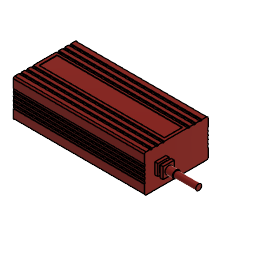
SSRHeatsink (Autodesk Fusion 360 archive; units mm, degrees)
design "BatteryCharger"
part number: 2026-09-24-16-56-48-668
Autodesk Fusion 360 part; units mm, degrees
note: some values were not read from the file. Set by a fixed rule: which face or edge a step refers to.
(part 1 of 3)
sketch "Sketch1" plane through (0, 0, 0) normal (0, 0, 1) x (1, 0, 0)
  line L0 (-87.5, 42.5) -> (87.5, 42.5)
  line L1 (87.5, 42.5) -> (87.5, -42.5)
  line L2 (87.5, -42.5) -> (-87.5, -42.5)
  line L3 (-87.5, -42.5) -> (-87.5, 42.5)
  line L4 (-87.5, 42.5) -> (87.5, -42.5) construction
  line L5 (87.5, 42.5) -> (-87.5, -42.5) construction
  dimension "d1" = 175
  dimension "d2" = 85
  constraint horizontal L0
  constraint perpendicular L0 L1
  constraint parallel L0 L2
  constraint parallel L1 L3
  constraint coincident L4 origin
  constraint coincident L5 origin
  measures "d1" distance of L1.end L2.end
  measures "d2" distance of L0.end L1.end
extrude "Extrude1" add sketch "Sketch1" along normal blind 50
sketch "Sketch2" plane through (0, 0, 50) normal (0, 0, 1) x (-1, 0, 0)
  line L0 (87.5, 42.5) -> (-87.5, 42.5)
  line L1 (-87.5, 42.5) -> (-87.5, -42.5)
  line L2 (-87.5, -42.5) -> (87.5, -42.5)
  line L3 (87.5, -42.5) -> (87.5, 42.5)
  line L4 (87.5, -15) -> (-87.5, -15)
  line L5 (-87.5, -15) -> (-87.5, 15)
  line L6 (-87.5, 15) -> (87.5, 15)
  line L7 (87.5, 15) -> (87.5, -15)
  line L8 (87.5, -15) -> (-87.5, 15) construction
  line L9 (-87.5, -15) -> (87.5, 15) construction
  line L10 (87.5, -15) -> (-87.5, -15)
  line L11 (-87.5, -15) -> (-87.5, -18)
  line L12 (-87.5, -18) -> (87.5, -18)
  line L13 (87.5, -18) -> (87.5, -15)
  line L14 (87.5, -18) -> (-87.5, -18)
  line L15 (-87.5, -18) -> (-87.5, -23)
  line L16 (-87.5, -23) -> (87.5, -23)
  line L17 (87.5, -23) -> (87.5, -18)
  line L18 (87.5, -23) -> (-87.5, -23)
  line L19 (-87.5, -23) -> (-87.5, -26)
  line L20 (-87.5, -26) -> (87.5, -26)
  line L21 (87.5, -26) -> (87.5, -23)
  line L22 (87.5, -26) -> (-87.5, -26)
  line L23 (-87.5, -26) -> (-87.5, -31)
  line L24 (-87.5, -31) -> (87.5, -31)
  line L25 (87.5, -31) -> (87.5, -26)
  line L26 (87.5, -31) -> (-87.5, -31)
  line L27 (-87.5, -31) -> (-87.5, -34)
  line L28 (-87.5, -34) -> (87.5, -34)
  line L29 (87.5, -34) -> (87.5, -31)
  dimension "d5" = 30
  dimension "d6" = 3
  dimension "d7" = 5
  dimension "d8" = 3
  dimension "d9" = 5
  dimension "d10" = 3
  constraint horizontal L4
  constraint perpendicular L4 L5
  constraint parallel L4 L6
  constraint parallel L5 L7
  constraint coincident L8 origin
  constraint coincident L9 origin
  constraint horizontal L10
  constraint vertical L11
  constraint horizontal L12
  constraint vertical L13
  constraint horizontal L14
  constraint vertical L15
  constraint horizontal L16
  constraint vertical L17
  constraint horizontal L18
  constraint vertical L19
  constraint horizontal L20
  constraint vertical L21
  constraint horizontal L22
  constraint vertical L23
  constraint horizontal L24
  constraint vertical L25
  constraint horizontal L26
  constraint vertical L27
  constraint horizontal L28
  constraint vertical L29
  measures "d5" distance of L4.end L5.end
  measures "d6" distance of L4.start L12.end
  measures "d7" distance of L12.end L16.end
  measures "d8" distance of L16.end L20.end
  measures "d9" distance of L20.end L24.end
  measures "d10" distance of L24.end L28.end
extrude "Extrude2" cut sketch "Sketch2" against normal blind 0.5 contours L1 L3 L4 L10 L11 L12 L13 L14 | L1 L3 L16 L18 L19 L20 L21 L22 | L1 L3 L24 L26 L27 L28 L29
fillet "Fillet1" radius 0.5 3 faces at (29.1667, 32, 49.5) (29.1667, 25, 49.5) (-29.1667, 16, 49.5)
pattern_linear "R-Pattern1" count 1 spacing 0 along (1, 0, 0) count 2 spacing 50 along (0, -1, 0) of "Extrude2", "Fillet1"
sketch "Sketch3" plane through (0, 0, 50) normal (0, 0, 1) x (-1, 0, 0)
  line L0 (87.5, 16) -> (87, 16)
  line L1 (87, 16) -> (-87, 16)
  line L2 (-87, 16) -> (-87.5, 16)
  line L3 (-87.5, 16) -> (-87.5, -15)
  line L4 (-87.5, -15) -> (-87, -15)
  line L5 (-87, -15) -> (87, -15)
  line L6 (87, -15) -> (87.5, -15)
  line L7 (87.5, -15) -> (87.5, 16)
  line L8 (83.4341, -11.9471) -> (-83.4341, -11.9471)
  line L9 (-83.4341, -11.9471) -> (-83.4341, 11.9471)
  line L10 (-83.4341, 11.9471) -> (83.4341, 11.9471)
  line L11 (83.4341, 11.9471) -> (83.4341, -11.9471)
  line L12 (83.4341, -11.9471) -> (-83.4341, 11.9471) construction
  line L13 (-83.4341, -11.9471) -> (83.4341, 11.9471) construction
  constraint horizontal L8
  constraint perpendicular L8 L9
  constraint parallel L8 L10
  constraint parallel L9 L11
  constraint coincident L12 origin
  constraint coincident L13 origin
extrude "Extrude3" cut sketch "Sketch3" against normal blind 0.5 contours L8 L9 L10 L11
sketch "Sketch4" plane through (0, -42.5, 0) normal (0, -1, 0) x (1, 0, 0)
  line L0 (-87.5, 0) -> (87.5, 0)
  line L1 (87.5, 0) -> (87.5, 50)
  line L2 (87.5, 50) -> (-87.5, 50)
  line L3 (-87.5, 50) -> (-87.5, 0)
  line L4 (0, 50) -> (0, 0) construction
  line L5 (-87.5, 26.5) -> (87.5, 26.5)
  line L6 (87.5, 26.5) -> (87.5, 23.5)
  line L7 (87.5, 23.5) -> (-87.5, 23.5)
  line L8 (-87.5, 23.5) -> (-87.5, 26.5)
  line L9 (-87.5, 26.5) -> (87.5, 23.5) construction
  line L10 (87.5, 26.5) -> (-87.5, 23.5) construction
  point P0 (0, 25)
  dimension "d21" = 3
  constraint midpoint L2 L4.start
  constraint coincident L4.end origin
  constraint horizontal L5
  constraint perpendicular L5 L6
  constraint parallel L5 L7
  constraint parallel L6 L8
  constraint coincident L9 P0
  constraint coincident L10 P0
  constraint midpoint L4 P0
  measures "d21" distance of L5.end L6.end
extrude "Extrude4" cut sketch "Sketch4" against normal blind 0.5 contours L1 L3 L5 L6 L7 L8
pattern_linear "R-Pattern2" count 1 spacing 0 along (-1, 0, 0) count 5 spacing 5 along (0, 0, 1) both ways of "Extrude4"
pattern_linear "R-Pattern3" count 1 spacing 0 along (0, 0, -1) count 2 spacing 84.5 along (0, 1, 0) of "Extrude4", "R-Pattern2"
fillet "Fillet2" radius 2 4 edges at (0, 42.5, 50) (0, 42.5, 0) (0, -42.5, 0) (0, -42.5, 50)
sketch "Sketch5" plane through (-87.5, 0, 0) normal (-1, 0, 0) x (0, -1, 0)
  arc A0 (42.5, 48) -> (40.5, 50) centre (40.5, 48) ccw
  line L0 (40.5, 50) -> (35, 50)
  line L1 (35, 50) -> (35, 49.866)
  spline S0 degree 3 poles (34.5, 49) (34.6385, 49.1385) (34.802, 49.3076) (34.9552, 49.5924) (35, 49.7386) (35, 49.866) knots 0 0 0 0 0.058781 0.058781 0.097013 0.097013 0.097013 0.097013
  line L2 (34.5, 49) -> (32.5, 49)
  spline S1 degree 3 poles (32, 49.866) (32, 49.7386) (32.0448, 49.5924) (32.198, 49.3076) (32.3615, 49.1385) (32.5, 49) knots 0.252766 0.252766 0.252766 0.252766 0.290998 0.290998 0.349779 0.349779 0.349779 0.349779
  line L3 (32, 49.866) -> (32, 50)
  line L4 (32, 50) -> (27, 50)
  line L5 (27, 50) -> (27, 49.866)
  spline S2 degree 3 poles (26.5, 49) (26.6385, 49.1385) (26.802, 49.3076) (26.9552, 49.5924) (27, 49.7386) (27, 49.866) knots 0 0 0 0 0.058781 0.058781 0.097013 0.097013 0.097013 0.097013
  line L6 (26.5, 49) -> (24.5, 49)
  spline S3 degree 3 poles (24, 49.866) (24, 49.7386) (24.0448, 49.5924) (24.198, 49.3076) (24.3615, 49.1385) (24.5, 49) knots 0.252766 0.252766 0.252766 0.252766 0.290998 0.290998 0.349779 0.349779 0.349779 0.349779
  line L7 (24, 49.866) -> (24, 50)
  line L8 (24, 50) -> (19, 50)
  line L9 (19, 50) -> (19, 49.866)
  spline S4 degree 3 poles (18.5, 49) (18.6385, 49.1385) (18.802, 49.3076) (18.9552, 49.5924) (19, 49.7386) (19, 49.866) knots 0 0 0 0 0.058781 0.058781 0.097013 0.097013 0.097013 0.097013
  line L10 (18.5, 49) -> (16.5, 49)
  spline S5 degree 3 poles (16, 49.866) (16, 49.7386) (16.0448, 49.5924) (16.198, 49.3076) (16.3615, 49.1385) (16.5, 49) knots 0.252766 0.252766 0.252766 0.252766 0.290998 0.290998 0.349779 0.349779 0.349779 0.349779
  line L11 (16, 49.866) -> (16, 50)
  line L12 (16, 50) -> (-15, 50)
  line L13 (-15, 50) -> (-15, 49.866)
  spline S6 degree 3 poles (-15.5, 49) (-15.3615, 49.1385) (-15.198, 49.3076) (-15.0448, 49.5924) (-15, 49.7386) (-15, 49.866) knots 0 0 0 0 0.058781 0.058781 0.097013 0.097013 0.097013 0.097013
  line L14 (-15.5, 49) -> (-17.5, 49)
  spline S7 degree 3 poles (-18, 49.866) (-18, 49.7386) (-17.9552, 49.5924) (-17.802, 49.3076) (-17.6385, 49.1385) (-17.5, 49) knots 0.252766 0.252766 0.252766 0.252766 0.290998 0.290998 0.349779 0.349779 0.349779 0.349779
  line L15 (-18, 49.866) -> (-18, 50)
  line L16 (-18, 50) -> (-23, 50)
  line L17 (-23, 50) -> (-23, 49.866)
  spline S8 degree 3 poles (-23.5, 49) (-23.3615, 49.1385) (-23.198, 49.3076) (-23.0448, 49.5924) (-23, 49.7386) (-23, 49.866) knots 0 0 0 0 0.058781 0.058781 0.097013 0.097013 0.097013 0.097013
  line L18 (-23.5, 49) -> (-25.5, 49)
  spline S9 degree 3 poles (-26, 49.866) (-26, 49.7386) (-25.9552, 49.5924) (-25.802, 49.3076) (-25.6385, 49.1385) (-25.5, 49) knots 0.252766 0.252766 0.252766 0.252766 0.290998 0.290998 0.349779 0.349779 0.349779 0.349779
  line L19 (-26, 49.866) -> (-26, 50)
  line L20 (-26, 50) -> (-31, 50)
  line L21 (-31, 50) -> (-31, 49.866)
  spline S10 degree 3 poles (-31.5, 49) (-31.3615, 49.1385) (-31.198, 49.3076) (-31.0448, 49.5924) (-31, 49.7386) (-31, 49.866) knots 0 0 0 0 0.058781 0.058781 0.097013 0.097013 0.097013 0.097013
  line L22 (-31.5, 49) -> (-33.5, 49)
  spline S11 degree 3 poles (-34, 49.866) (-34, 49.7386) (-33.9552, 49.5924) (-33.802, 49.3076) (-33.6385, 49.1385) (-33.5, 49) knots 0.252766 0.252766 0.252766 0.252766 0.290998 0.290998 0.349779 0.349779 0.349779 0.349779
  line L23 (-34, 49.866) -> (-34, 50)
  line L24 (-34, 50) -> (-40.5, 50)
  arc A1 (-40.5, 50) -> (-42.5, 48) centre (-40.5, 48) ccw
  line L25 (-42.5, 48) -> (-42.5, 36.5)
  line L26 (-42.5, 36.5) -> (-42, 36.5)
  line L27 (-42, 36.5) -> (-42, 33.5)
  line L28 (-42, 33.5) -> (-42.5, 33.5)
  line L29 (-42.5, 33.5) -> (-42.5, 31.5)
  line L30 (-42.5, 31.5) -> (-42, 31.5)
  line L31 (-42, 31.5) -> (-42, 28.5)
  line L32 (-42, 28.5) -> (-42.5, 28.5)
  line L33 (-42.5, 28.5) -> (-42.5, 26.5)
  line L34 (-42.5, 26.5) -> (-42, 26.5)
  line L35 (-42, 26.5) -> (-42, 23.5)
  line L36 (-42, 23.5) -> (-42.5, 23.5)
  line L37 (-42.5, 23.5) -> (-42.5, 21.5)
  line L38 (-42.5, 21.5) -> (-42, 21.5)
  line L39 (-42, 21.5) -> (-42, 18.5)
  line L40 (-42, 18.5) -> (-42.5, 18.5)
  line L41 (-42.5, 18.5) -> (-42.5, 16.5)
  line L42 (-42.5, 16.5) -> (-42, 16.5)
  line L43 (-42, 16.5) -> (-42, 13.5)
  line L44 (-42, 13.5) -> (-42.5, 13.5)
  line L45 (-42.5, 13.5) -> (-42.5, 2)
  arc A2 (-42.5, 2) -> (-40.5, 0) centre (-40.5, 2) ccw
  line L46 (-40.5, 0) -> (40.5, 0)
  arc A3 (40.5, 0) -> (42.5, 2) centre (40.5, 2) ccw
  line L47 (42.5, 2) -> (42.5, 13.5)
  line L48 (42.5, 13.5) -> (42, 13.5)
  line L49 (42, 13.5) -> (42, 16.5)
  line L50 (42, 16.5) -> (42.5, 16.5)
  line L51 (42.5, 16.5) -> (42.5, 18.5)
  line L52 (42.5, 18.5) -> (42, 18.5)
  line L53 (42, 18.5) -> (42, 21.5)
  line L54 (42, 21.5) -> (42.5, 21.5)
  line L55 (42.5, 21.5) -> (42.5, 23.5)
  line L56 (42.5, 23.5) -> (42, 23.5)
  line L57 (42, 23.5) -> (42, 26.5)
  line L58 (42, 26.5) -> (42.5, 26.5)
  line L59 (42.5, 26.5) -> (42.5, 28.5)
  line L60 (42.5, 28.5) -> (42, 28.5)
  line L61 (42, 28.5) -> (42, 31.5)
  line L62 (42, 31.5) -> (42.5, 31.5)
  line L63 (42.5, 31.5) -> (42.5, 33.5)
  line L64 (42.5, 33.5) -> (42, 33.5)
  line L65 (42, 33.5) -> (42, 36.5)
  line L66 (42, 36.5) -> (42.5, 36.5)
  line L67 (42.5, 36.5) -> (42.5, 48)
  line L68 (-41.9142, 49.4142) -> (41.9142, 0.5858) construction
  line L69 (-38.5, 45.5) -> (38.5, 45.5) construction
  line L70 (38.5, 45.5) -> (38.5, 4.5) construction
  line L71 (38.5, 4.5) -> (-38.5, 4.5) construction
  line L72 (-38.5, 4.5) -> (-38.5, 45.5) construction
  line L73 (-38.5, 45.5) -> (38.5, 4.5) construction
  line L74 (38.5, 45.5) -> (-38.5, 4.5) construction
  circle A4 centre (-38.5, 45.5) radius 1.5
  circle A5 centre (38.5, 45.5) radius 1.5
  circle A6 centre (-38.5, 4.5) radius 1.5
  circle A7 centre (38.5, 4.5) radius 1.5
  point P0 (0, 25)
  dimension "d34" = 77
  dimension "d35" = 41
  dimension "d36" = 3
  dimension "d37" = 3
  dimension "d38" = 3
  dimension "d39" = 3
  constraint midpoint A1 L68.start
  constraint midpoint A3 L68.end
  constraint horizontal L69
  constraint perpendicular L69 L70
  constraint parallel L69 L71
  constraint parallel L70 L72
  constraint coincident L73 P0
  constraint coincident L74 P0
  constraint midpoint L68 P0
  constraint coincident L69.start L72.end
  constraint coincident L69.end L70.start
  constraint coincident L71.end L72.start
  constraint coincident L70.end L71.start
  measures "d34" distance of L70.end L71.end
  measures "d35" distance of L69.end L70.end
  measures "d36" diameter of A4
  measures "d37" diameter of A5
  measures "d38" diameter of A6
  measures "d39" diameter of A7
extrude "Extrude5" add sketch "Sketch5" along normal blind 2 contours A4 | A5 | A6 | A7
fillet "Fillet3" radius 0.5 4 edges at (-89.5, 39.8985, 44.9576) (-89.5, 39.8985, 3.9576) (-89.5, -37.1015, 44.9576) (-89.5, -37.1015, 3.9576)
sketch "Sketch6" plane through (-87.5, 0, 0) normal (-1, 0, 0) x (0, -1, 0)
  circle A0 centre (38.5, 4.5) radius 1.5
  circle A1 centre (-38.5, 45.5) radius 1.5
  circle A2 centre (38.5, 45.5) radius 1.5
  circle A3 centre (-38.5, 4.5) radius 1.5
  arc A4 (42.5, 48) -> (40.5, 50) centre (40.5, 48) ccw
  line L0 (40.5, 50) -> (35, 50)
  line L1 (35, 50) -> (35, 49.866)
  spline S0 degree 3 poles (34.5, 49) (34.6385, 49.1385) (34.802, 49.3076) (34.9552, 49.5924) (35, 49.7386) (35, 49.866) knots 0 0 0 0 0.058781 0.058781 0.097013 0.097013 0.097013 0.097013
  line L2 (34.5, 49) -> (32.5, 49)
  spline S1 degree 3 poles (32, 49.866) (32, 49.7386) (32.0448, 49.5924) (32.198, 49.3076) (32.3615, 49.1385) (32.5, 49) knots 0.252766 0.252766 0.252766 0.252766 0.290998 0.290998 0.349779 0.349779 0.349779 0.349779
  line L3 (32, 49.866) -> (32, 50)
  line L4 (32, 50) -> (27, 50)
  line L5 (27, 50) -> (27, 49.866)
  spline S2 degree 3 poles (26.5, 49) (26.6385, 49.1385) (26.802, 49.3076) (26.9552, 49.5924) (27, 49.7386) (27, 49.866) knots 0 0 0 0 0.058781 0.058781 0.097013 0.097013 0.097013 0.097013
  line L6 (26.5, 49) -> (24.5, 49)
  spline S3 degree 3 poles (24, 49.866) (24, 49.7386) (24.0448, 49.5924) (24.198, 49.3076) (24.3615, 49.1385) (24.5, 49) knots 0.252766 0.252766 0.252766 0.252766 0.290998 0.290998 0.349779 0.349779 0.349779 0.349779
  line L7 (24, 49.866) -> (24, 50)
  line L8 (24, 50) -> (19, 50)
  line L9 (19, 50) -> (19, 49.866)
  spline S4 degree 3 poles (18.5, 49) (18.6385, 49.1385) (18.802, 49.3076) (18.9552, 49.5924) (19, 49.7386) (19, 49.866) knots 0 0 0 0 0.058781 0.058781 0.097013 0.097013 0.097013 0.097013
  line L10 (18.5, 49) -> (16.5, 49)
  spline S5 degree 3 poles (16, 49.866) (16, 49.7386) (16.0448, 49.5924) (16.198, 49.3076) (16.3615, 49.1385) (16.5, 49) knots 0.252766 0.252766 0.252766 0.252766 0.290998 0.290998 0.349779 0.349779 0.349779 0.349779
  line L11 (16, 49.866) -> (16, 50)
  line L12 (16, 50) -> (-15, 50)
  line L13 (-15, 50) -> (-15, 49.866)
  spline S6 degree 3 poles (-15.5, 49) (-15.3615, 49.1385) (-15.198, 49.3076) (-15.0448, 49.5924) (-15, 49.7386) (-15, 49.866) knots 0 0 0 0 0.058781 0.058781 0.097013 0.097013 0.097013 0.097013
  line L14 (-15.5, 49) -> (-17.5, 49)
  spline S7 degree 3 poles (-18, 49.866) (-18, 49.7386) (-17.9552, 49.5924) (-17.802, 49.3076) (-17.6385, 49.1385) (-17.5, 49) knots 0.252766 0.252766 0.252766 0.252766 0.290998 0.290998 0.349779 0.349779 0.349779 0.349779
  line L15 (-18, 49.866) -> (-18, 50)
  line L16 (-18, 50) -> (-23, 50)
  line L17 (-23, 50) -> (-23, 49.866)
  spline S8 degree 3 poles (-23.5, 49) (-23.3615, 49.1385) (-23.198, 49.3076) (-23.0448, 49.5924) (-23, 49.7386) (-23, 49.866) knots 0 0 0 0 0.058781 0.058781 0.097013 0.097013 0.097013 0.097013
  line L18 (-23.5, 49) -> (-25.5, 49)
  spline S9 degree 3 poles (-26, 49.866) (-26, 49.7386) (-25.9552, 49.5924) (-25.802, 49.3076) (-25.6385, 49.1385) (-25.5, 49) knots 0.252766 0.252766 0.252766 0.252766 0.290998 0.290998 0.349779 0.349779 0.349779 0.349779
  line L19 (-26, 49.866) -> (-26, 50)
  line L20 (-26, 50) -> (-31, 50)
  line L21 (-31, 50) -> (-31, 49.866)
  spline S10 degree 3 poles (-31.5, 49) (-31.3615, 49.1385) (-31.198, 49.3076) (-31.0448, 49.5924) (-31, 49.7386) (-31, 49.866) knots 0 0 0 0 0.058781 0.058781 0.097013 0.097013 0.097013 0.097013
  line L22 (-31.5, 49) -> (-33.5, 49)
  spline S11 degree 3 poles (-34, 49.866) (-34, 49.7386) (-33.9552, 49.5924) (-33.802, 49.3076) (-33.6385, 49.1385) (-33.5, 49) knots 0.252766 0.252766 0.252766 0.252766 0.290998 0.290998 0.349779 0.349779 0.349779 0.349779
  line L23 (-34, 49.866) -> (-34, 50)
  line L24 (-34, 50) -> (-40.5, 50)
  arc A5 (-40.5, 50) -> (-42.5, 48) centre (-40.5, 48) ccw
  line L25 (-42.5, 48) -> (-42.5, 36.5)
  line L26 (-42.5, 36.5) -> (-42, 36.5)
  line L27 (-42, 36.5) -> (-42, 33.5)
  line L28 (-42, 33.5) -> (-42.5, 33.5)
  line L29 (-42.5, 33.5) -> (-42.5, 31.5)
  line L30 (-42.5, 31.5) -> (-42, 31.5)
  line L31 (-42, 31.5) -> (-42, 28.5)
  line L32 (-42, 28.5) -> (-42.5, 28.5)
  line L33 (-42.5, 28.5) -> (-42.5, 26.5)
  line L34 (-42.5, 26.5) -> (-42, 26.5)
  line L35 (-42, 26.5) -> (-42, 23.5)
  line L36 (-42, 23.5) -> (-42.5, 23.5)
  line L37 (-42.5, 23.5) -> (-42.5, 21.5)
  line L38 (-42.5, 21.5) -> (-42, 21.5)
  line L39 (-42, 21.5) -> (-42, 18.5)
  line L40 (-42, 18.5) -> (-42.5, 18.5)
  line L41 (-42.5, 18.5) -> (-42.5, 16.5)
  line L42 (-42.5, 16.5) -> (-42, 16.5)
  line L43 (-42, 16.5) -> (-42, 13.5)
  line L44 (-42, 13.5) -> (-42.5, 13.5)
  line L45 (-42.5, 13.5) -> (-42.5, 2)
  arc A6 (-42.5, 2) -> (-40.5, 0) centre (-40.5, 2) ccw
  line L46 (-40.5, 0) -> (40.5, 0)
  arc A7 (40.5, 0) -> (42.5, 2) centre (40.5, 2) ccw
  line L47 (42.5, 2) -> (42.5, 13.5)
  line L48 (42.5, 13.5) -> (42, 13.5)
  line L49 (42, 13.5) -> (42, 16.5)
  line L50 (42, 16.5) -> (42.5, 16.5)
  line L51 (42.5, 16.5) -> (42.5, 18.5)
  line L52 (42.5, 18.5) -> (42, 18.5)
  line L53 (42, 18.5) -> (42, 21.5)
  line L54 (42, 21.5) -> (42.5, 21.5)
  line L55 (42.5, 21.5) -> (42.5, 23.5)
  line L56 (42.5, 23.5) -> (42, 23.5)
  line L57 (42, 23.5) -> (42, 26.5)
  line L58 (42, 26.5) -> (42.5, 26.5)
  line L59 (42.5, 26.5) -> (42.5, 28.5)
  line L60 (42.5, 28.5) -> (42, 28.5)
  line L61 (42, 28.5) -> (42, 31.5)
  line L62 (42, 31.5) -> (42.5, 31.5)
  line L63 (42.5, 31.5) -> (42.5, 33.5)
  line L64 (42.5, 33.5) -> (42, 33.5)
  line L65 (42, 33.5) -> (42, 36.5)
  line L66 (42, 36.5) -> (42.5, 36.5)
  line L67 (42.5, 36.5) -> (42.5, 48)
  line L68 (42, 25) -> (0, 25) construction
  line L69 (21, 25) -> (-42, 25) construction
  circle A8 centre (-10.5, 25) radius 17.5
  circle A9 centre (-10.5, 25) radius 15
  circle A10 centre (-10.5, 25) radius 12.5
  circle A11 centre (-10.5, 25) radius 10
  circle A12 centre (-10.5, 25) radius 7.5
  line L70 (-9.5, 46.0108) -> (-11.5, 46.0108)
  line L71 (-11.5, 46.0108) -> (-11.5, 3.9892)
  line L72 (-11.5, 3.9892) -> (-9.5, 3.9892)
  line L73 (-9.5, 3.9892) -> (-9.5, 46.0108)
  line L74 (-9.5, 46.0108) -> (-11.5, 3.9892) construction
  line L75 (-11.5, 46.0108) -> (-9.5, 3.9892) construction
  line L76 (15, 26) -> (-36, 26)
  line L77 (-36, 26) -> (-36, 24)
  line L78 (-36, 24) -> (15, 24)
  line L79 (15, 24) -> (15, 26)
  line L80 (15, 26) -> (-36, 24) construction
  line L81 (-36, 26) -> (15, 24) construction
  point P0 (-10.5, 25)
  point P1 (-10.5, 25)
  dimension "d44" = 35
  dimension "d45" = 30
  dimension "d46" = 25
  dimension "d47" = 20
  dimension "d48" = 15
  dimension "d49" = 2
  dimension "d50" = 51
  dimension "d51" = 2
  constraint midpoint L57 L68.start
  constraint perpendicular L57 L68
  constraint midpoint L68 L69.start
  constraint midpoint L35 L69.end
  constraint midpoint L69 P1
  constraint concentric A8 A9
  constraint concentric A8 A10
  constraint concentric A9 A11
  constraint concentric A8 A12
  constraint horizontal L70
  constraint perpendicular L70 L71
  constraint parallel L70 L72
  constraint parallel L71 L73
  constraint coincident L74 P1
  constraint coincident L75 P1
  constraint coincident P1 P0
  constraint horizontal L76
  constraint perpendicular L76 L77
  constraint parallel L76 L78
  constraint parallel L77 L79
  constraint coincident L80 P1
  constraint coincident L81 P1
  measures "d44" diameter of A8
  measures "d45" diameter of A9
  measures "d46" diameter of A10
  measures "d47" diameter of A11
  measures "d48" diameter of A12
  measures "d49" distance of L71.end L72.end
  measures "d50" distance of L77.end L78.end
  measures "d51" distance of L76.end L77.end
extrude "Extrude6" cut sketch "Sketch6" against normal blind 5 contours A8 A9 L73 L76 | A8 A9 L73 L78 | A8 A9 L71 L76 | A10 A11 L73 L76 | A8 A9 L71 L78 | A10 A11 L73 L78 | A10 A11 L71 L76 | A10 A11 L71 L78
sketch "Sketch7" plane through (-87.5, 0, 0) normal (-1, 0, 0) x (0, -1, 0)
  arc A0 (42.5, 48) -> (40.5, 50) centre (40.5, 48) ccw
  line L0 (40.5, 50) -> (35, 50)
  line L1 (35, 50) -> (35, 49.866)
  spline S0 degree 3 poles (34.5, 49) (34.6385, 49.1385) (34.802, 49.3076) (34.9552, 49.5924) (35, 49.7386) (35, 49.866) knots 0 0 0 0 0.058781 0.058781 0.097013 0.097013 0.097013 0.097013
  line L2 (34.5, 49) -> (32.5, 49)
  spline S1 degree 3 poles (32, 49.866) (32, 49.7386) (32.0448, 49.5924) (32.198, 49.3076) (32.3615, 49.1385) (32.5, 49) knots 0.252766 0.252766 0.252766 0.252766 0.290998 0.290998 0.349779 0.349779 0.349779 0.349779
  line L3 (32, 49.866) -> (32, 50)
  line L4 (32, 50) -> (27, 50)
  line L5 (27, 50) -> (27, 49.866)
  spline S2 degree 3 poles (26.5, 49) (26.6385, 49.1385) (26.802, 49.3076) (26.9552, 49.5924) (27, 49.7386) (27, 49.866) knots 0 0 0 0 0.058781 0.058781 0.097013 0.097013 0.097013 0.097013
  line L6 (26.5, 49) -> (24.5, 49)
  spline S3 degree 3 poles (24, 49.866) (24, 49.7386) (24.0448, 49.5924) (24.198, 49.3076) (24.3615, 49.1385) (24.5, 49) knots 0.252766 0.252766 0.252766 0.252766 0.290998 0.290998 0.349779 0.349779 0.349779 0.349779
  line L7 (24, 49.866) -> (24, 50)
  line L8 (24, 50) -> (19, 50)
  line L9 (19, 50) -> (19, 49.866)
  spline S4 degree 3 poles (18.5, 49) (18.6385, 49.1385) (18.802, 49.3076) (18.9552, 49.5924) (19, 49.7386) (19, 49.866) knots 0 0 0 0 0.058781 0.058781 0.097013 0.097013 0.097013 0.097013
  line L10 (18.5, 49) -> (16.5, 49)
  spline S5 degree 3 poles (16, 49.866) (16, 49.7386) (16.0448, 49.5924) (16.198, 49.3076) (16.3615, 49.1385) (16.5, 49) knots 0.252766 0.252766 0.252766 0.252766 0.290998 0.290998 0.349779 0.349779 0.349779 0.349779
  line L11 (16, 49.866) -> (16, 50)
  line L12 (16, 50) -> (-15, 50)
  line L13 (-15, 50) -> (-15, 49.866)
  spline S6 degree 3 poles (-15.5, 49) (-15.3615, 49.1385) (-15.198, 49.3076) (-15.0448, 49.5924) (-15, 49.7386) (-15, 49.866) knots 0 0 0 0 0.058781 0.058781 0.097013 0.097013 0.097013 0.097013
  line L14 (-15.5, 49) -> (-17.5, 49)
  spline S7 degree 3 poles (-18, 49.866) (-18, 49.7386) (-17.9552, 49.5924) (-17.802, 49.3076) (-17.6385, 49.1385) (-17.5, 49) knots 0.252766 0.252766 0.252766 0.252766 0.290998 0.290998 0.349779 0.349779 0.349779 0.349779
  line L15 (-18, 49.866) -> (-18, 50)
  line L16 (-18, 50) -> (-23, 50)
  line L17 (-23, 50) -> (-23, 49.866)
  spline S8 degree 3 poles (-23.5, 49) (-23.3615, 49.1385) (-23.198, 49.3076) (-23.0448, 49.5924) (-23, 49.7386) (-23, 49.866) knots 0 0 0 0 0.058781 0.058781 0.097013 0.097013 0.097013 0.097013
  line L18 (-23.5, 49) -> (-25.5, 49)
  spline S9 degree 3 poles (-26, 49.866) (-26, 49.7386) (-25.9552, 49.5924) (-25.802, 49.3076) (-25.6385, 49.1385) (-25.5, 49) knots 0.252766 0.252766 0.252766 0.252766 0.290998 0.290998 0.349779 0.349779 0.349779 0.349779
  line L19 (-26, 49.866) -> (-26, 50)
  line L20 (-26, 50) -> (-31, 50)
  line L21 (-31, 50) -> (-31, 49.866)
  spline S10 degree 3 poles (-31.5, 49) (-31.3615, 49.1385) (-31.198, 49.3076) (-31.0448, 49.5924) (-31, 49.7386) (-31, 49.866) knots 0 0 0 0 0.058781 0.058781 0.097013 0.097013 0.097013 0.097013
  line L22 (-31.5, 49) -> (-33.5, 49)
  spline S11 degree 3 poles (-34, 49.866) (-34, 49.7386) (-33.9552, 49.5924) (-33.802, 49.3076) (-33.6385, 49.1385) (-33.5, 49) knots 0.252766 0.252766 0.252766 0.252766 0.290998 0.290998 0.349779 0.349779 0.349779 0.349779
  line L23 (-34, 49.866) -> (-34, 50)
  line L24 (-34, 50) -> (-40.5, 50)
  arc A1 (-40.5, 50) -> (-42.5, 48) centre (-40.5, 48) ccw
  line L25 (-42.5, 48) -> (-42.5, 36.5)
  line L26 (-42.5, 36.5) -> (-42, 36.5)
  line L27 (-42, 36.5) -> (-42, 33.5)
  line L28 (-42, 33.5) -> (-42.5, 33.5)
  line L29 (-42.5, 33.5) -> (-42.5, 31.5)
  line L30 (-42.5, 31.5) -> (-42, 31.5)
  line L31 (-42, 31.5) -> (-42, 28.5)
  line L32 (-42, 28.5) -> (-42.5, 28.5)
  line L33 (-42.5, 28.5) -> (-42.5, 26.5)
  line L34 (-42.5, 26.5) -> (-42, 26.5)
  line L35 (-42, 26.5) -> (-42, 23.5)
  line L36 (-42, 23.5) -> (-42.5, 23.5)
  line L37 (-42.5, 23.5) -> (-42.5, 21.5)
  line L38 (-42.5, 21.5) -> (-42, 21.5)
  line L39 (-42, 21.5) -> (-42, 18.5)
  line L40 (-42, 18.5) -> (-42.5, 18.5)
  line L41 (-42.5, 18.5) -> (-42.5, 16.5)
  line L42 (-42.5, 16.5) -> (-42, 16.5)
  line L43 (-42, 16.5) -> (-42, 13.5)
  line L44 (-42, 13.5) -> (-42.5, 13.5)
  line L45 (-42.5, 13.5) -> (-42.5, 2)
  arc A2 (-42.5, 2) -> (-40.5, 0) centre (-40.5, 2) ccw
  line L46 (-40.5, 0) -> (40.5, 0)
  arc A3 (40.5, 0) -> (42.5, 2) centre (40.5, 2) ccw
  line L47 (42.5, 2) -> (42.5, 13.5)
  line L48 (42.5, 13.5) -> (42, 13.5)
  line L49 (42, 13.5) -> (42, 16.5)
  line L50 (42, 16.5) -> (42.5, 16.5)
  line L51 (42.5, 16.5) -> (42.5, 18.5)
  line L52 (42.5, 18.5) -> (42, 18.5)
  line L53 (42, 18.5) -> (42, 21.5)
  line L54 (42, 21.5) -> (42.5, 21.5)
  line L55 (42.5, 21.5) -> (42.5, 23.5)
  line L56 (42.5, 23.5) -> (42, 23.5)
  line L57 (42, 23.5) -> (42, 26.5)
  line L58 (42, 26.5) -> (42.5, 26.5)
  line L59 (42.5, 26.5) -> (42.5, 28.5)
  line L60 (42.5, 28.5) -> (42, 28.5)
  line L61 (42, 28.5) -> (42, 31.5)
  line L62 (42, 31.5) -> (42.5, 31.5)
  line L63 (42.5, 31.5) -> (42.5, 33.5)
  line L64 (42.5, 33.5) -> (42, 33.5)
  line L65 (42, 33.5) -> (42, 36.5)
  line L66 (42, 36.5) -> (42.5, 36.5)
  line L67 (42.5, 36.5) -> (42.5, 48)
  circle A4 centre (-38.5, 4.5) radius 1.5
  circle A5 centre (38.5, 45.5) radius 1.5
  circle A6 centre (-38.5, 45.5) radius 1.5
  circle A7 centre (38.5, 4.5) radius 1.5
  arc A8 (-22.9599, 24) -> (-11.5, 12.5401) centre (-10.5, 25) ccw
  line L68 (-22.9599, 24) -> (-20.4499, 24)
  arc A9 (-20.4499, 24) -> (-11.5, 15.0501) centre (-10.5, 25) ccw
  line L69 (-11.5, 15.0501) -> (-11.5, 12.5401)
  arc A10 (-27.9714, 24) -> (-11.5, 7.5286) centre (-10.5, 25) ccw
  line L70 (-27.9714, 24) -> (-25.4666, 24)
  arc A11 (-25.4666, 24) -> (-11.5, 10.0334) centre (-10.5, 25) ccw
  line L71 (-11.5, 10.0334) -> (-11.5, 7.5286)
  arc A12 (-11.5, 42.4714) -> (-27.9714, 26) centre (-10.5, 25) ccw
  line L72 (-11.5, 42.4714) -> (-11.5, 39.9666)
  arc A13 (-11.5, 39.9666) -> (-25.4666, 26) centre (-10.5, 25) ccw
  line L73 (-25.4666, 26) -> (-27.9714, 26)
  arc A14 (-11.5, 37.4599) -> (-22.9599, 26) centre (-10.5, 25) ccw
  line L74 (-11.5, 37.4599) -> (-11.5, 34.9499)
  arc A15 (-11.5, 34.9499) -> (-20.4499, 26) centre (-10.5, 25) ccw
  line L75 (-20.4499, 26) -> (-22.9599, 26)
  arc A16 (-9.5, 12.5401) -> (1.9599, 24) centre (-10.5, 25) ccw
  line L76 (-9.5, 12.5401) -> (-9.5, 15.0501)
  arc A17 (-9.5, 15.0501) -> (-0.5501, 24) centre (-10.5, 25) ccw
  line L77 (-0.5501, 24) -> (1.9599, 24)
  arc A18 (-9.5, 7.5286) -> (6.9714, 24) centre (-10.5, 25) ccw
  line L78 (-9.5, 7.5286) -> (-9.5, 10.0334)
  arc A19 (-9.5, 10.0334) -> (4.4666, 24) centre (-10.5, 25) ccw
  line L79 (4.4666, 24) -> (6.9714, 24)
  arc A20 (6.9714, 26) -> (-9.5, 42.4714) centre (-10.5, 25) ccw
  line L80 (6.9714, 26) -> (4.4666, 26)
  arc A21 (4.4666, 26) -> (-9.5, 39.9666) centre (-10.5, 25) ccw
  line L81 (-9.5, 39.9666) -> (-9.5, 42.4714)
  arc A22 (1.9599, 26) -> (-9.5, 37.4599) centre (-10.5, 25) ccw
  line L82 (1.9599, 26) -> (-0.5501, 26)
  arc A23 (-0.5501, 26) -> (-9.5, 34.9499) centre (-10.5, 25) ccw
  line L83 (-9.5, 34.9499) -> (-9.5, 37.4599)
  line L84 (14, 37) -> (30, 37)
  line L85 (30, 37) -> (30, 13)
  line L86 (30, 13) -> (14, 13)
  line L87 (14, 13) -> (14, 37)
  line L88 (14, 37) -> (30, 13) construction
  line L89 (30, 37) -> (14, 13) construction
  point P0 (22, 25)
  dimension "d54" = 16
  dimension "d55" = 24
  constraint horizontal L84
  constraint perpendicular L84 L85
  constraint parallel L84 L86
  constraint parallel L85 L87
  constraint coincident L88 P0
  constraint coincident L89 P0
  measures "d54" distance of L85.end L86.end
  measures "d55" distance of L84.end L85.end
extrude "Extrude7" cut sketch "Sketch7" against normal blind 10 contours L84 L85 L86 L87
chamfer "Chamfer1" distance 5 distance2 5 2 edges at (-82.5, -30, 37) (-82.5, -30, 13) measured on face at (-84.1667, -30, 29) measured on face at (-80.8333, -24.6667, 13)
fillet "Fillet4" radius 2 2 edges at (-82.5, -14, 37) (-82.5, -14, 13)
sketch "Sketch8" plane through (-87.5, 0, 0) normal (-1, 0, 0) x (0, -1, 0)
  arc A0 (1.9599, 26) -> (-9.5, 37.4599) centre (-10.5, 25) ccw
  line L0 (1.9599, 26) -> (-0.5501, 26)
  arc A1 (-0.5501, 26) -> (-9.5, 34.9499) centre (-10.5, 25) ccw
  line L1 (-9.5, 34.9499) -> (-9.5, 37.4599)
  arc A2 (6.9714, 26) -> (-9.5, 42.4714) centre (-10.5, 25) ccw
  line L2 (6.9714, 26) -> (4.4666, 26)
  arc A3 (4.4666, 26) -> (-9.5, 39.9666) centre (-10.5, 25) ccw
  line L3 (-9.5, 39.9666) -> (-9.5, 42.4714)
  arc A4 (-9.5, 7.5286) -> (6.9714, 24) centre (-10.5, 25) ccw
  line L4 (-9.5, 7.5286) -> (-9.5, 10.0334)
  arc A5 (-9.5, 10.0334) -> (4.4666, 24) centre (-10.5, 25) ccw
  line L5 (4.4666, 24) -> (6.9714, 24)
  arc A6 (-9.5, 12.5401) -> (1.9599, 24) centre (-10.5, 25) ccw
  line L6 (-9.5, 12.5401) -> (-9.5, 15.0501)
  arc A7 (-9.5, 15.0501) -> (-0.5501, 24) centre (-10.5, 25) ccw
  line L7 (-0.5501, 24) -> (1.9599, 24)
  arc A8 (-11.5, 37.4599) -> (-22.9599, 26) centre (-10.5, 25) ccw
  line L8 (-11.5, 37.4599) -> (-11.5, 34.9499)
  arc A9 (-11.5, 34.9499) -> (-20.4499, 26) centre (-10.5, 25) ccw
  line L9 (-20.4499, 26) -> (-22.9599, 26)
  arc A10 (-11.5, 42.4714) -> (-27.9714, 26) centre (-10.5, 25) ccw
  line L10 (-11.5, 42.4714) -> (-11.5, 39.9666)
  arc A11 (-11.5, 39.9666) -> (-25.4666, 26) centre (-10.5, 25) ccw
  line L11 (-25.4666, 26) -> (-27.9714, 26)
  arc A12 (-27.9714, 24) -> (-11.5, 7.5286) centre (-10.5, 25) ccw
  line L12 (-27.9714, 24) -> (-25.4666, 24)
  arc A13 (-25.4666, 24) -> (-11.5, 10.0334) centre (-10.5, 25) ccw
  line L13 (-11.5, 10.0334) -> (-11.5, 7.5286)
  arc A14 (-22.9599, 24) -> (-11.5, 12.5401) centre (-10.5, 25) ccw
  line L14 (-22.9599, 24) -> (-20.4499, 24)
  arc A15 (-20.4499, 24) -> (-11.5, 15.0501) centre (-10.5, 25) ccw
  line L15 (-11.5, 15.0501) -> (-11.5, 12.5401)
  circle A16 centre (38.5, 4.5) radius 1.5
  circle A17 centre (-38.5, 45.5) radius 1.5
  circle A18 centre (38.5, 45.5) radius 1.5
  circle A19 centre (-38.5, 4.5) radius 1.5
  arc A20 (42.5, 48) -> (40.5, 50) centre (40.5, 48) ccw
  line L16 (40.5, 50) -> (35, 50)
  line L17 (35, 50) -> (35, 49.866)
  spline S0 degree 3 poles (34.5, 49) (34.6385, 49.1385) (34.802, 49.3076) (34.9552, 49.5924) (35, 49.7386) (35, 49.866) knots 0 0 0 0 0.058781 0.058781 0.097013 0.097013 0.097013 0.097013
  line L18 (34.5, 49) -> (32.5, 49)
  spline S1 degree 3 poles (32, 49.866) (32, 49.7386) (32.0448, 49.5924) (32.198, 49.3076) (32.3615, 49.1385) (32.5, 49) knots 0.252766 0.252766 0.252766 0.252766 0.290998 0.290998 0.349779 0.349779 0.349779 0.349779
  line L19 (32, 49.866) -> (32, 50)
  line L20 (32, 50) -> (27, 50)
  line L21 (27, 50) -> (27, 49.866)
  spline S2 degree 3 poles (26.5, 49) (26.6385, 49.1385) (26.802, 49.3076) (26.9552, 49.5924) (27, 49.7386) (27, 49.866) knots 0 0 0 0 0.058781 0.058781 0.097013 0.097013 0.097013 0.097013
  line L22 (26.5, 49) -> (24.5, 49)
  spline S3 degree 3 poles (24, 49.866) (24, 49.7386) (24.0448, 49.5924) (24.198, 49.3076) (24.3615, 49.1385) (24.5, 49) knots 0.252766 0.252766 0.252766 0.252766 0.290998 0.290998 0.349779 0.349779 0.349779 0.349779
  line L23 (24, 49.866) -> (24, 50)
  line L24 (24, 50) -> (19, 50)
  line L25 (19, 50) -> (19, 49.866)
  spline S4 degree 3 poles (18.5, 49) (18.6385, 49.1385) (18.802, 49.3076) (18.9552, 49.5924) (19, 49.7386) (19, 49.866) knots 0 0 0 0 0.058781 0.058781 0.097013 0.097013 0.097013 0.097013
  line L26 (18.5, 49) -> (16.5, 49)
  spline S5 degree 3 poles (16, 49.866) (16, 49.7386) (16.0448, 49.5924) (16.198, 49.3076) (16.3615, 49.1385) (16.5, 49) knots 0.252766 0.252766 0.252766 0.252766 0.290998 0.290998 0.349779 0.349779 0.349779 0.349779
  line L27 (16, 49.866) -> (16, 50)
  line L28 (16, 50) -> (-15, 50)
  line L29 (-15, 50) -> (-15, 49.866)
  spline S6 degree 3 poles (-15.5, 49) (-15.3615, 49.1385) (-15.198, 49.3076) (-15.0448, 49.5924) (-15, 49.7386) (-15, 49.866) knots 0 0 0 0 0.058781 0.058781 0.097013 0.097013 0.097013 0.097013
  line L30 (-15.5, 49) -> (-17.5, 49)
  spline S7 degree 3 poles (-18, 49.866) (-18, 49.7386) (-17.9552, 49.5924) (-17.802, 49.3076) (-17.6385, 49.1385) (-17.5, 49) knots 0.252766 0.252766 0.252766 0.252766 0.290998 0.290998 0.349779 0.349779 0.349779 0.349779
  line L31 (-18, 49.866) -> (-18, 50)
  line L32 (-18, 50) -> (-23, 50)
  line L33 (-23, 50) -> (-23, 49.866)
  spline S8 degree 3 poles (-23.5, 49) (-23.3615, 49.1385) (-23.198, 49.3076) (-23.0448, 49.5924) (-23, 49.7386) (-23, 49.866) knots 0 0 0 0 0.058781 0.058781 0.097013 0.097013 0.097013 0.097013
  line L34 (-23.5, 49) -> (-25.5, 49)
  spline S9 degree 3 poles (-26, 49.866) (-26, 49.7386) (-25.9552, 49.5924) (-25.802, 49.3076) (-25.6385, 49.1385) (-25.5, 49) knots 0.252766 0.252766 0.252766 0.252766 0.290998 0.290998 0.349779 0.349779 0.349779 0.349779
  line L35 (-26, 49.866) -> (-26, 50)
  line L36 (-26, 50) -> (-31, 50)
  line L37 (-31, 50) -> (-31, 49.866)
  spline S10 degree 3 poles (-31.5, 49) (-31.3615, 49.1385) (-31.198, 49.3076) (-31.0448, 49.5924) (-31, 49.7386) (-31, 49.866) knots 0 0 0 0 0.058781 0.058781 0.097013 0.097013 0.097013 0.097013
  line L38 (-31.5, 49) -> (-33.5, 49)
  spline S11 degree 3 poles (-34, 49.866) (-34, 49.7386) (-33.9552, 49.5924) (-33.802, 49.3076) (-33.6385, 49.1385) (-33.5, 49) knots 0.252766 0.252766 0.252766 0.252766 0.290998 0.290998 0.349779 0.349779 0.349779 0.349779
  line L39 (-34, 49.866) -> (-34, 50)
  line L40 (-34, 50) -> (-40.5, 50)
  arc A21 (-40.5, 50) -> (-42.5, 48) centre (-40.5, 48) ccw
  line L41 (-42.5, 48) -> (-42.5, 36.5)
  line L42 (-42.5, 36.5) -> (-42, 36.5)
  line L43 (-42, 36.5) -> (-42, 33.5)
  line L44 (-42, 33.5) -> (-42.5, 33.5)
  line L45 (-42.5, 33.5) -> (-42.5, 31.5)
  line L46 (-42.5, 31.5) -> (-42, 31.5)
  line L47 (-42, 31.5) -> (-42, 28.5)
  line L48 (-42, 28.5) -> (-42.5, 28.5)
  line L49 (-42.5, 28.5) -> (-42.5, 26.5)
  line L50 (-42.5, 26.5) -> (-42, 26.5)
  line L51 (-42, 26.5) -> (-42, 23.5)
  line L52 (-42, 23.5) -> (-42.5, 23.5)
  line L53 (-42.5, 23.5) -> (-42.5, 21.5)
  line L54 (-42.5, 21.5) -> (-42, 21.5)
  line L55 (-42, 21.5) -> (-42, 18.5)
  line L56 (-42, 18.5) -> (-42.5, 18.5)
  line L57 (-42.5, 18.5) -> (-42.5, 16.5)
  line L58 (-42.5, 16.5) -> (-42, 16.5)
  line L59 (-42, 16.5) -> (-42, 13.5)
  line L60 (-42, 13.5) -> (-42.5, 13.5)
  line L61 (-42.5, 13.5) -> (-42.5, 2)
  arc A22 (-42.5, 2) -> (-40.5, 0) centre (-40.5, 2) ccw
  line L62 (-40.5, 0) -> (40.5, 0)
  arc A23 (40.5, 0) -> (42.5, 2) centre (40.5, 2) ccw
  line L63 (42.5, 2) -> (42.5, 13.5)
  line L64 (42.5, 13.5) -> (42, 13.5)
  line L65 (42, 13.5) -> (42, 16.5)
  line L66 (42, 16.5) -> (42.5, 16.5)
  line L67 (42.5, 16.5) -> (42.5, 18.5)
  line L68 (42.5, 18.5) -> (42, 18.5)
  line L69 (42, 18.5) -> (42, 21.5)
  line L70 (42, 21.5) -> (42.5, 21.5)
  line L71 (42.5, 21.5) -> (42.5, 23.5)
  line L72 (42.5, 23.5) -> (42, 23.5)
  line L73 (42, 23.5) -> (42, 26.5)
  line L74 (42, 26.5) -> (42.5, 26.5)
  line L75 (42.5, 26.5) -> (42.5, 28.5)
  line L76 (42.5, 28.5) -> (42, 28.5)
  line L77 (42, 28.5) -> (42, 31.5)
  line L78 (42, 31.5) -> (42.5, 31.5)
  line L79 (42.5, 31.5) -> (42.5, 33.5)
  line L80 (42.5, 33.5) -> (42, 33.5)
  line L81 (42, 33.5) -> (42, 36.5)
  line L82 (42, 36.5) -> (42.5, 36.5)
  line L83 (42.5, 36.5) -> (42.5, 48)
  line L84 (30, 32) -> (30, 18)
  line L85 (30, 18) -> (25, 13)
  line L86 (25, 13) -> (16, 13)
  arc A24 (14, 15) -> (16, 13) centre (16, 15) ccw
  line L87 (14, 15) -> (14, 35)
  arc A25 (16, 37) -> (14, 35) centre (16, 35) ccw
  line L88 (16, 37) -> (25, 37)
  line L89 (25, 37) -> (30, 32)
  line L90 (30, 25) -> (14, 25) construction
  line L91 (12, 39) -> (32, 39)
  line L92 (32, 39) -> (32, 11)
  line L93 (32, 11) -> (12, 11)
  line L94 (12, 11) -> (12, 39)
  line L95 (12, 39) -> (32, 11) construction
  line L96 (32, 39) -> (12, 11) construction
  point P0 (22, 25)
  dimension "d62" = 20
  dimension "d63" = 28
  constraint midpoint L84 L90.start
  constraint midpoint L87 L90.end
  constraint horizontal L91
  constraint perpendicular L91 L92
  constraint parallel L91 L93
  constraint parallel L92 L94
  constraint coincident L95 P0
  constraint coincident L96 P0
  constraint midpoint L90 P0
  measures "d62" distance of L92.end L93.end
  measures "d63" distance of L91.end L92.end
extrude "Extrude8" add sketch "Sketch8" along normal blind 4 contours L91 L92 L93 L94
sketch "Sketch9" plane through (-87.5, 0, 0) normal (-1, 0, 0) x (0, -1, 0)
  arc A0 (42.5, 48) -> (40.5, 50) centre (40.5, 48) ccw
  line L0 (40.5, 50) -> (35, 50)
  line L1 (35, 50) -> (35, 49.866)
  spline S0 degree 3 poles (34.5, 49) (34.6385, 49.1385) (34.802, 49.3076) (34.9552, 49.5924) (35, 49.7386) (35, 49.866) knots 0 0 0 0 0.058781 0.058781 0.097013 0.097013 0.097013 0.097013
  line L2 (34.5, 49) -> (32.5, 49)
  spline S1 degree 3 poles (32, 49.866) (32, 49.7386) (32.0448, 49.5924) (32.198, 49.3076) (32.3615, 49.1385) (32.5, 49) knots 0.252766 0.252766 0.252766 0.252766 0.290998 0.290998 0.349779 0.349779 0.349779 0.349779
  line L3 (32, 49.866) -> (32, 50)
  line L4 (32, 50) -> (27, 50)
  line L5 (27, 50) -> (27, 49.866)
  spline S2 degree 3 poles (26.5, 49) (26.6385, 49.1385) (26.802, 49.3076) (26.9552, 49.5924) (27, 49.7386) (27, 49.866) knots 0 0 0 0 0.058781 0.058781 0.097013 0.097013 0.097013 0.097013
  line L6 (26.5, 49) -> (24.5, 49)
  spline S3 degree 3 poles (24, 49.866) (24, 49.7386) (24.0448, 49.5924) (24.198, 49.3076) (24.3615, 49.1385) (24.5, 49) knots 0.252766 0.252766 0.252766 0.252766 0.290998 0.290998 0.349779 0.349779 0.349779 0.349779
  line L7 (24, 49.866) -> (24, 50)
  line L8 (24, 50) -> (19, 50)
  line L9 (19, 50) -> (19, 49.866)
  spline S4 degree 3 poles (18.5, 49) (18.6385, 49.1385) (18.802, 49.3076) (18.9552, 49.5924) (19, 49.7386) (19, 49.866) knots 0 0 0 0 0.058781 0.058781 0.097013 0.097013 0.097013 0.097013
  line L10 (18.5, 49) -> (16.5, 49)
  spline S5 degree 3 poles (16, 49.866) (16, 49.7386) (16.0448, 49.5924) (16.198, 49.3076) (16.3615, 49.1385) (16.5, 49) knots 0.252766 0.252766 0.252766 0.252766 0.290998 0.290998 0.349779 0.349779 0.349779 0.349779
  line L11 (16, 49.866) -> (16, 50)
  line L12 (16, 50) -> (-15, 50)
  line L13 (-15, 50) -> (-15, 49.866)
  spline S6 degree 3 poles (-15.5, 49) (-15.3615, 49.1385) (-15.198, 49.3076) (-15.0448, 49.5924) (-15, 49.7386) (-15, 49.866) knots 0 0 0 0 0.058781 0.058781 0.097013 0.097013 0.097013 0.097013
  line L14 (-15.5, 49) -> (-17.5, 49)
  spline S7 degree 3 poles (-18, 49.866) (-18, 49.7386) (-17.9552, 49.5924) (-17.802, 49.3076) (-17.6385, 49.1385) (-17.5, 49) knots 0.252766 0.252766 0.252766 0.252766 0.290998 0.290998 0.349779 0.349779 0.349779 0.349779
  line L15 (-18, 49.866) -> (-18, 50)
  line L16 (-18, 50) -> (-23, 50)
  line L17 (-23, 50) -> (-23, 49.866)
  spline S8 degree 3 poles (-23.5, 49) (-23.3615, 49.1385) (-23.198, 49.3076) (-23.0448, 49.5924) (-23, 49.7386) (-23, 49.866) knots 0 0 0 0 0.058781 0.058781 0.097013 0.097013 0.097013 0.097013
  line L18 (-23.5, 49) -> (-25.5, 49)
  spline S9 degree 3 poles (-26, 49.866) (-26, 49.7386) (-25.9552, 49.5924) (-25.802, 49.3076) (-25.6385, 49.1385) (-25.5, 49) knots 0.252766 0.252766 0.252766 0.252766 0.290998 0.290998 0.349779 0.349779 0.349779 0.349779
  line L19 (-26, 49.866) -> (-26, 50)
  line L20 (-26, 50) -> (-31, 50)
  line L21 (-31, 50) -> (-31, 49.866)
  spline S10 degree 3 poles (-31.5, 49) (-31.3615, 49.1385) (-31.198, 49.3076) (-31.0448, 49.5924) (-31, 49.7386) (-31, 49.866) knots 0 0 0 0 0.058781 0.058781 0.097013 0.097013 0.097013 0.097013
  line L22 (-31.5, 49) -> (-33.5, 49)
  spline S11 degree 3 poles (-34, 49.866) (-34, 49.7386) (-33.9552, 49.5924) (-33.802, 49.3076) (-33.6385, 49.1385) (-33.5, 49) knots 0.252766 0.252766 0.252766 0.252766 0.290998 0.290998 0.349779 0.349779 0.349779 0.349779
  line L23 (-34, 49.866) -> (-34, 50)
  line L24 (-34, 50) -> (-40.5, 50)
  arc A1 (-40.5, 50) -> (-42.5, 48) centre (-40.5, 48) ccw
  line L25 (-42.5, 48) -> (-42.5, 36.5)
  line L26 (-42.5, 36.5) -> (-42, 36.5)
  line L27 (-42, 36.5) -> (-42, 33.5)
  line L28 (-42, 33.5) -> (-42.5, 33.5)
  line L29 (-42.5, 33.5) -> (-42.5, 31.5)
  line L30 (-42.5, 31.5) -> (-42, 31.5)
  line L31 (-42, 31.5) -> (-42, 28.5)
  line L32 (-42, 28.5) -> (-42.5, 28.5)
  line L33 (-42.5, 28.5) -> (-42.5, 26.5)
  line L34 (-42.5, 26.5) -> (-42, 26.5)
  line L35 (-42, 26.5) -> (-42, 23.5)
  line L36 (-42, 23.5) -> (-42.5, 23.5)
  line L37 (-42.5, 23.5) -> (-42.5, 21.5)
  line L38 (-42.5, 21.5) -> (-42, 21.5)
  line L39 (-42, 21.5) -> (-42, 18.5)
  line L40 (-42, 18.5) -> (-42.5, 18.5)
  line L41 (-42.5, 18.5) -> (-42.5, 16.5)
  line L42 (-42.5, 16.5) -> (-42, 16.5)
  line L43 (-42, 16.5) -> (-42, 13.5)
  line L44 (-42, 13.5) -> (-42.5, 13.5)
  line L45 (-42.5, 13.5) -> (-42.5, 2)
  arc A2 (-42.5, 2) -> (-40.5, 0) centre (-40.5, 2) ccw
  line L46 (-40.5, 0) -> (40.5, 0)
  arc A3 (40.5, 0) -> (42.5, 2) centre (40.5, 2) ccw
  line L47 (42.5, 2) -> (42.5, 13.5)
  line L48 (42.5, 13.5) -> (42, 13.5)
  line L49 (42, 13.5) -> (42, 16.5)
  line L50 (42, 16.5) -> (42.5, 16.5)
  line L51 (42.5, 16.5) -> (42.5, 18.5)
  line L52 (42.5, 18.5) -> (42, 18.5)
  line L53 (42, 18.5) -> (42, 21.5)
  line L54 (42, 21.5) -> (42.5, 21.5)
  line L55 (42.5, 21.5) -> (42.5, 23.5)
  line L56 (42.5, 23.5) -> (42, 23.5)
  line L57 (42, 23.5) -> (42, 26.5)
  line L58 (42, 26.5) -> (42.5, 26.5)
  line L59 (42.5, 26.5) -> (42.5, 28.5)
  line L60 (42.5, 28.5) -> (42, 28.5)
  line L61 (42, 28.5) -> (42, 31.5)
  line L62 (42, 31.5) -> (42.5, 31.5)
  line L63 (42.5, 31.5) -> (42.5, 33.5)
  line L64 (42.5, 33.5) -> (42, 33.5)
  line L65 (42, 33.5) -> (42, 36.5)
  line L66 (42, 36.5) -> (42.5, 36.5)
  line L67 (42.5, 36.5) -> (42.5, 48)
  circle A4 centre (-38.5, 4.5) radius 1.5
  circle A5 centre (38.5, 45.5) radius 1.5
  circle A6 centre (-38.5, 45.5) radius 1.5
  circle A7 centre (38.5, 4.5) radius 1.5
  arc A8 (-22.9599, 24) -> (-11.5, 12.5401) centre (-10.5, 25) ccw
  line L68 (-22.9599, 24) -> (-20.4499, 24)
  arc A9 (-20.4499, 24) -> (-11.5, 15.0501) centre (-10.5, 25) ccw
  line L69 (-11.5, 15.0501) -> (-11.5, 12.5401)
  arc A10 (-27.9714, 24) -> (-11.5, 7.5286) centre (-10.5, 25) ccw
  line L70 (-27.9714, 24) -> (-25.4666, 24)
  arc A11 (-25.4666, 24) -> (-11.5, 10.0334) centre (-10.5, 25) ccw
  line L71 (-11.5, 10.0334) -> (-11.5, 7.5286)
  arc A12 (-11.5, 42.4714) -> (-27.9714, 26) centre (-10.5, 25) ccw
  line L72 (-11.5, 42.4714) -> (-11.5, 39.9666)
  arc A13 (-11.5, 39.9666) -> (-25.4666, 26) centre (-10.5, 25) ccw
  line L73 (-25.4666, 26) -> (-27.9714, 26)
  arc A14 (-11.5, 37.4599) -> (-22.9599, 26) centre (-10.5, 25) ccw
  line L74 (-11.5, 37.4599) -> (-11.5, 34.9499)
  arc A15 (-11.5, 34.9499) -> (-20.4499, 26) centre (-10.5, 25) ccw
  line L75 (-20.4499, 26) -> (-22.9599, 26)
  arc A16 (-9.5, 12.5401) -> (1.9599, 24) centre (-10.5, 25) ccw
  line L76 (-9.5, 12.5401) -> (-9.5, 15.0501)
  arc A17 (-9.5, 15.0501) -> (-0.5501, 24) centre (-10.5, 25) ccw
  line L77 (-0.5501, 24) -> (1.9599, 24)
  arc A18 (-9.5, 7.5286) -> (6.9714, 24) centre (-10.5, 25) ccw
  line L78 (-9.5, 7.5286) -> (-9.5, 10.0334)
  arc A19 (-9.5, 10.0334) -> (4.4666, 24) centre (-10.5, 25) ccw
  line L79 (4.4666, 24) -> (6.9714, 24)
  arc A20 (6.9714, 26) -> (-9.5, 42.4714) centre (-10.5, 25) ccw
  line L80 (6.9714, 26) -> (4.4666, 26)
  arc A21 (4.4666, 26) -> (-9.5, 39.9666) centre (-10.5, 25) ccw
  line L81 (-9.5, 39.9666) -> (-9.5, 42.4714)
  arc A22 (1.9599, 26) -> (-9.5, 37.4599) centre (-10.5, 25) ccw
  line L82 (1.9599, 26) -> (-0.5501, 26)
  arc A23 (-0.5501, 26) -> (-9.5, 34.9499) centre (-10.5, 25) ccw
  line L83 (-9.5, 34.9499) -> (-9.5, 37.4599)
  line L84 (12, 11) -> (12, 39)
  line L85 (12, 39) -> (32, 39)
  line L86 (32, 39) -> (32, 11)
  line L87 (32, 11) -> (12, 11)
  line L88 (22, 39) -> (22, 45)
  line L89 (22, 11) -> (22, 5)
  line L90 (19.942, 43.7652) -> (12, 39)
  line L91 (24.058, 43.7652) -> (32, 39)
  line L92 (24.058, 6.2348) -> (32, 11)
  line L93 (19.942, 6.2348) -> (12, 11)
  arc A24 (24.058, 43.7652) -> (19.942, 43.7652) centre (22, 40.3352) ccw
  arc A25 (19.942, 6.2348) -> (24.058, 6.2348) centre (22, 9.6648) ccw
  dimension "d66" = 6
  dimension "d67" = 4
  constraint midpoint L85 L88.start
  constraint perpendicular L85 L88
  constraint midpoint L87 L89.start
  constraint perpendicular L87 L89
  constraint coincident L84.end L85.start
  constraint coincident L85.end L86.start
  constraint coincident L86.end L87.start
  constraint coincident L84.start L87.end
  constraint coincident L88.end L91
  constraint coincident L88.end L90
  constraint tangent L91 A24
  constraint tangent L90 A24
  constraint coincident L89.end L92
  constraint coincident L89.end L93
  constraint tangent L92 A25
  constraint tangent L93 A25
  constraint equal A24 A25
  measures "d66" distance of L89.start L89.end
  measures "d67" radius of A24
extrude "Extrude9" add sketch "Sketch9" along normal blind 3 contours L87 L89 L93 A25 | L85 L88 L90 A24 | L87 L89 L92 A25 | L85 L88 L91 A24
sketch "Sketch10" plane through (-90.5, 0, 0) normal (-1, 0, 0) x (0, -1, 0)
  arc A0 (24.058, 43.7652) -> (19.942, 43.7652) centre (22, 40.3352) ccw
  line L0 (19.942, 43.7652) -> (12, 39)
  line L1 (12, 39) -> (32, 39)
  line L2 (32, 39) -> (24.058, 43.7652)
  line L3 (22, 44.3352) -> (22, 39) construction
  circle A1 centre (22, 41.6676) radius 1.5
  dimension "d70" = 3
  constraint midpoint A0 L3.start
  constraint midpoint L1 L3.end
  constraint midpoint L3 A1.centre
  measures "d70" diameter of A1
extrude "Extrude10" add sketch "Sketch10" along normal blind 2 contours A1
fillet "Fillet5" radius 0.5 1 edges at (-92.5, -20.6015, 41.1252)
pattern_linear "R-Pattern4" count 1 spacing 0 along (0, 1, 0) count 2 spacing 33 along (0, 0, -1) of "Extrude10", "Fillet5"
fillet "Fillet6" radius 2 8 edges at (-89, -32, 39) (-91, -32, 39) (-91, -12, 39) (-89, -12, 39) (-91, -12, 11) (-89, -12, 11) (-89, -32, 11) (-91, -32, 11)